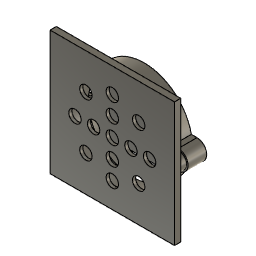
Speaker+Mount+Rev+1 (Autodesk Fusion 360 design; units mm, degrees)
Autodesk Fusion 360 part; units mm, degrees
sketch "Face" plane through (0, 0, 0) normal (0, 1, 0) x (1, 0, 0)
  line L0 (0, 0) -> (40, 0)
  line L1 (40, 0) -> (40, -40)
  line L2 (40, -40) -> (0, -40)
  line L3 (0, -40) -> (0, 0)
  circle A0 centre (20, -20) radius 14
  circle A1 centre (20, -20) radius 14.2
  circle A2 centre (20, -20) radius 14.7
  line L4 (0, -20) -> (40, -20)
  line L5 (5.5141, -22.5) -> (0.5141, -22.5)
  line L6 (0.5141, -22.5) -> (0.5141, -17.5)
  line L7 (0.5141, -17.5) -> (5.5141, -17.5)
  line L8 (5.5141, -17.5) -> (5.5141, -22.5)
  circle A3 centre (3.0141, -20) radius 2.5
  circle A4 centre (3.0141, -20) radius 1.5
  line L9 (34.4859, -22.5) -> (39.4859, -22.5)
  line L10 (39.4859, -22.5) -> (39.4859, -17.5)
  line L11 (39.4859, -17.5) -> (34.4859, -17.5)
  line L12 (34.4859, -17.5) -> (34.4859, -22.5)
  circle A5 centre (36.9859, -20) radius 2.5
  circle A6 centre (36.9859, -20) radius 1.5
  circle A7 centre (20, -32) radius 2
  circle A8 centre (28.4853, -28.4853) radius 2
  circle A9 centre (32, -20) radius 2
  circle A10 centre (28.4853, -11.5147) radius 2
  circle A11 centre (20, -8) radius 2
  circle A12 centre (11.5147, -11.5147) radius 2
  circle A13 centre (8, -20) radius 2
  circle A14 centre (11.5147, -28.4853) radius 2
  circle A15 centre (20, -26) radius 2
  circle A16 centre (26, -20) radius 2
  circle A17 centre (20, -14) radius 2
  circle A18 centre (14, -20) radius 2
  circle A19 centre (20, -20) radius 2
  dimension "d1" = 40
  dimension "d2" = 40
  dimension "d3" = 28
  dimension "d21" = 28.4
  dimension "d22" = 29.4
  dimension "d31" = 20
  dimension "d32" = 20
  dimension "d33" = 5
  dimension "d34" = 5
  dimension "d35" = 2.5
  dimension "d36" = 5
  dimension "d37" = 2.5
  dimension "d38" = 3
  dimension "d39" = 5
  dimension "d41" = 2.5
  dimension "d42" = 5
  dimension "d43" = 2.5
  dimension "d44" = 3
  dimension "d62" = 4
  dimension "d63" = 12
  dimension "d65" = 360
  dimension "d66" = 4
  dimension "d67" = 6
  dimension "d69" = 360
  dimension "d70" = 4
  constraint horizontal L0
  constraint vertical L1
  constraint horizontal L2
  constraint vertical L3
  constraint coincident L0.start L3.end
  constraint midpoint L3 L4.start
  constraint midpoint L1 L4.end
  constraint horizontal L5
  constraint vertical L6
  constraint horizontal L7
  constraint vertical L8
  constraint coincident A2 L5.start
  constraint coincident L4 A3.centre
  constraint concentric A3 A4
  constraint horizontal L9
  constraint vertical L10
  constraint horizontal L11
  constraint vertical L12
  constraint coincident A2 L9.start
  constraint coincident L4 A5.centre
  constraint concentric A5 A6
  constraint concentric A0 A19
  measures "d1" distance of L0.start L0.end
  measures "d2" distance of L0.start L2.end
  measures "d3" diameter of A0
  measures "d21" diameter of A1
  measures "d22" diameter of A2
  measures "d31" distance of L3 A0.centre
  measures "d32" distance of L0 A0.centre
  measures "d33" distance of L5.start L5.end
  measures "d34" distance of L5.start L7.end
  measures "d35" distance of L4 L7
  measures "d36" diameter of A3
  measures "d37" distance of L6 A3.centre
  measures "d38" diameter of A4
  measures "d39" distance of L9.start L9.end
  measures "d41" distance of L4 L9
  measures "d42" diameter of A5
  measures "d43" distance of L10 A5.centre
  measures "d44" diameter of A6
  measures "d62" diameter of A7
  measures "d63" distance of A0.centre A7.centre
  measures "d66" diameter of A15
  measures "d67" distance of A0.centre A15.centre
  measures "d70" diameter of A19
extrude "Extrude1" add sketch "Face" along normal blind 2 contours L0 L1 L3 A2 L4 L6 L7 L10 L11 | L1 L2 L3 A2 L4 L5 L6 L9 L10 | A2 L4 A3 A4 | L5 L6 A3 | L6 L7 A3 | A2 L4 A3 A4 | A2 L4 A5 A6 | L10 L11 A5 | A2 L4 A5 A6 | L9 L10 A5 | L4 A4 | L4 A4 | A2 L7 A3 | A2 L5 A3 | L4 A6 | L4 A6 | A2 L11 A5 | A2 L9 A5 makes body 1
extrude "Extrude2" add sketch "Face" along normal blind 6 contours A2 L8 A3 | A1 A2 L4 L8 L12 | A2 L4 A3 | A1 A2 L4 L8 L12 | A2 L8 A3 | A2 L4 A3 | A2 L12 A5 | A2 L4 A5 | A2 L12 A5 | A2 L4 A5 bodies 1
extrude "Extrude3" add sketch "Face" along normal blind 1 contours A0 A1 L4 | A0 A1 L4 | A14 | A7 | A8 | A0 L4 A9 A13 A16 A18 A19 | L4 A13 | A10 | A11 | A12 | A0 L4 A9 A13 A16 A18 A19 | L4 A13 | L4 A9 | L4 A9 | L4 A18 | L4 A18 | L4 A16 | L4 A16 | L4 A19 | L4 A19 | A15 | A17 bodies 1
extrude "Extrude4" add 1 faces at (5.5214, 6, 20.7303) along direction (0, 1, 0) blind 0.5 on bodies 1 bodies 1
extrude "Extrude5" add sketch "Face" along normal blind 6.5 contours A2 L4 A3 A4 | A2 L4 A3 A4 | A2 L4 A5 A6 | A2 L4 A5 A6 | A2 L7 A3 | A2 L5 A3 | A2 L11 A5 | A2 L9 A5 bodies 1
sketch "Back" plane through (0, 6.5, 0) normal (0, 1, 0) x (-1, 0, 0)
  circle A0 centre (-36.9859, 20) radius 1.5
  circle A1 centre (-3.0141, 20) radius 1.5
  circle A2 centre (-20, 20) radius 14.2
  arc A3 (-5.5141, 22.5) -> (-34.4859, 22.5) centre (-20, 20) ccw
  line L0 (-34.4859, 22.5) -> (-36.9859, 22.5)
  arc A4 (-36.9859, 22.5) -> (-36.9859, 17.5) centre (-36.9859, 20) ccw
  line L1 (-36.9859, 17.5) -> (-34.4859, 17.5)
  arc A5 (-34.4859, 17.5) -> (-5.5141, 17.5) centre (-20, 20) ccw
  line L2 (-5.5141, 17.5) -> (-3.0141, 17.5)
  arc A6 (-3.0141, 17.5) -> (-3.0141, 22.5) centre (-3.0141, 20) ccw
  line L3 (-3.0141, 22.5) -> (-5.5141, 22.5)
  circle A7 centre (-20, 20) radius 15
  circle A8 centre (-20, 20) radius 15.5
  circle A9 centre (-3.0141, 20) radius 2.65
  circle A10 centre (-36.9859, 20) radius 2.65
  circle A11 centre (-36.9859, 20) radius 3.15
  circle A12 centre (-3.0141, 20) radius 3.15
  line L4 (-36.9859, 20) -> (-35.1765, 20)
  line L5 (-35.1765, 20) -> (-35.1765, 23.15)
  line L6 (-35.1765, 23.15) -> (-36.9859, 23.15)
  line L7 (-36.9859, 23.15) -> (-36.9859, 20)
  line L8 (-36.9859, 20) -> (-35.1765, 20)
  line L9 (-35.1765, 20) -> (-35.1765, 16.85)
  line L10 (-35.1765, 16.85) -> (-36.9859, 16.85)
  line L11 (-36.9859, 16.85) -> (-36.9859, 20)
  line L12 (-36.9859, 20) -> (-35.0233, 20)
  line L13 (-35.0233, 20) -> (-35.0233, 22.65)
  line L14 (-35.0233, 22.65) -> (-36.9859, 22.65)
  line L15 (-36.9859, 22.65) -> (-36.9859, 20)
  line L16 (-36.9859, 17.35) -> (-35.1765, 17.35)
  line L17 (-35.1765, 17.35) -> (-35.1765, 20)
  line L18 (-35.1765, 20) -> (-36.9859, 20)
  line L19 (-36.9859, 20) -> (-36.9859, 17.35)
  line L20 (-3.0141, 23.15) -> (-5, 23.15)
  line L21 (-5, 23.15) -> (-5, 20)
  line L22 (-5, 20) -> (-3.0141, 20)
  line L23 (-3.0141, 20) -> (-3.0141, 23.15)
  line L24 (-3.0141, 22.65) -> (-5, 22.65)
  line L25 (-5, 22.65) -> (-5, 20)
  line L26 (-5, 20) -> (-3.0141, 20)
  line L27 (-3.0141, 20) -> (-3.0141, 22.65)
  line L28 (-3.0141, 16.85) -> (-5, 16.85)
  line L29 (-5, 16.85) -> (-5, 20)
  line L30 (-5, 20) -> (-3.0141, 20)
  line L31 (-3.0141, 20) -> (-3.0141, 16.85)
  line L32 (-5, 20) -> (-3.0141, 20)
  line L33 (-3.0141, 20) -> (-3.0141, 17.35)
  line L34 (-3.0141, 17.35) -> (-5, 17.35)
  line L35 (-5, 17.35) -> (-5, 20)
  line L36 (-35.1765, 17.35) -> (-34.6587, 17.35)
  line L37 (-34.6587, 17.35) -> (-34.6587, 16.8182)
  line L38 (-34.6587, 16.8182) -> (-35.1765, 16.8182)
  line L39 (-35.1765, 16.8182) -> (-35.1765, 17.35)
  line L40 (-35.0233, 22.65) -> (-34.6587, 22.65)
  line L41 (-34.6587, 22.65) -> (-34.6587, 23.1818)
  line L42 (-34.6587, 23.1818) -> (-35.0233, 23.1818)
  line L43 (-35.0233, 23.1818) -> (-35.0233, 22.65)
  line L44 (-5, 22.65) -> (-5.3413, 22.65)
  line L45 (-5.3413, 22.65) -> (-5.3413, 23.1818)
  line L46 (-5.3413, 23.1818) -> (-5, 23.1818)
  line L47 (-5, 23.1818) -> (-5, 22.65)
  line L48 (-5, 17.35) -> (-5.3413, 17.35)
  line L49 (-5.3413, 17.35) -> (-5.3413, 16.8182)
  line L50 (-5.3413, 16.8182) -> (-5, 16.8182)
  line L51 (-5, 16.8182) -> (-5, 17.35)
  dimension "d47" = 30
  dimension "d48" = 31
  dimension "d49" = 5.3
  dimension "d50" = 5.3
  dimension "d51" = 6.3
  dimension "d52" = 6.3
  dimension "d53" = 3.15
  dimension "d54" = 3.15
  dimension "d55" = 2.65
  constraint concentric A2 A7
  constraint concentric A7 A8
  constraint concentric A1 A9
  constraint concentric A0 A10
  constraint concentric A10 A11
  constraint concentric A9 A12
  constraint horizontal L4
  constraint vertical L5
  constraint horizontal L6
  constraint vertical L7
  constraint coincident A8 L5.end
  constraint coincident A0.centre A4.centre
  constraint horizontal L8
  constraint vertical L9
  constraint horizontal L10
  constraint vertical L11
  constraint coincident A8 L9.end
  constraint horizontal L12
  constraint vertical L13
  constraint horizontal L14
  constraint vertical L15
  constraint horizontal L16
  constraint vertical L17
  constraint horizontal L18
  constraint vertical L19
  constraint coincident L11 L16.start
  constraint coincident A10 L16.start
  constraint horizontal L20
  constraint vertical L21
  constraint horizontal L22
  constraint vertical L23
  constraint coincident A7 L21.end
  constraint coincident A12 L20.start
  constraint horizontal L24
  constraint vertical L25
  constraint horizontal L26
  constraint vertical L27
  constraint coincident A9 L24.start
  constraint coincident L23 L24.start
  constraint horizontal L28
  constraint vertical L29
  constraint horizontal L30
  constraint vertical L31
  constraint coincident A12 L28.start
  constraint horizontal L32
  constraint vertical L33
  constraint horizontal L34
  constraint vertical L35
  constraint coincident L31 L33.end
  constraint coincident A9 L33.end
  constraint horizontal L36
  constraint vertical L37
  constraint horizontal L38
  constraint vertical L39
  constraint coincident A7 L37.end
  constraint horizontal L40
  constraint vertical L41
  constraint horizontal L42
  constraint vertical L43
  constraint coincident A7 L41.end
  constraint horizontal L44
  constraint vertical L45
  constraint horizontal L46
  constraint vertical L47
  constraint coincident A7 L45.end
  constraint horizontal L48
  constraint vertical L49
  constraint horizontal L50
  constraint vertical L51
  constraint coincident A7 L49.end
  measures "d47" diameter of A7
  measures "d48" diameter of A8
  measures "d49" diameter of A9
  measures "d50" diameter of A10
  measures "d51" diameter of A11
  measures "d52" diameter of A12
  measures "d53" distance of A0.centre L6.end
  measures "d54" distance of A0.centre L10.end
  measures "d55" distance of A0.centre L14.end
extrude "Extrude6" add sketch "Back" against normal blind 1 separate body contours A0 A8 A10 L4 L8 L9 L12 L17 L18 | A0 A8 A10 L4 L5 L8 L12 L18 | A0 L0 A8 A10 L7 L15 | A0 L1 A8 A10 L11 L19 | A7 A10 L9 L12 L13 L17 | A10 L5 L12 L13 | A0 A4 L7 L11 L15 L19 | L0 A8 A10 | L0 A8 A10 L5 | L1 A8 A10 L9 L17 | L1 A8 A10 | L0 A10 A11 L5 L13 | L1 A7 A10 A11 L9 L17 | L0 A10 L7 L15 | A4 A10 L7 L11 L15 L19 | L0 A8 A11 L5 | L0 A8 A10 A11 L14 | L1 A10 L11 L19 | L1 A8 A10 A11 L16 | L1 A8 A11 L9 L17 | A7 A10 A11 L13 | L0 A11 L5 | A2 A7 A10 A11 | A7 A10 | L1 A11 L9 L17 | A10 A11 L7 L11 | A11 L7 L14 | A8 A11 L14 | A8 A11 L5 L14 | A11 L11 L16 | A8 A11 L9 L16 L17 | A8 A11 L16 | L0 A7 A11 L13 | L0 A11 L13 | L0 A11 L5 L13 L14 | A2 L1 A5 L2 A7 A11 A12 | L1 A7 A11 | L1 A7 A11 L9 L17 L36 | A8 A11 L6 L14 | A8 L5 L14 | A8 A11 L10 L16 | A8 L9 L16 L39 | A2 A3 L0 L3 A7 A11 A12 | L0 A7 L13 L40 | A7 A8 L5 L14 L20 L42 L43 L46 L47 | L1 A5 L2 A7 L36 L37 L48 L49 | A2 A11 A12 | A2 A11 | A7 A8 L9 L36 L38 L39 | A3 L0 L3 A7 L40 L41 L44 L45 | A7 L40 L42 L43 | A7 L36 L37 | A2 A12 | A2 A7 A9 A12 | A8 A12 L20 L24 | A8 L20 L21 L24 L47 | A7 A8 L28 L38 L50 L51 | A7 L40 L41 | L2 A7 A12 L29 L35 | A7 A9 A12 L29 L35 | A8 A12 L24 | L3 A8 A12 L21 L24 L25 | A12 L23 L24 | A9 A12 L23 L31 | A7 L21 L44 L46 L47 | A8 L28 L29 L34 L51 | A8 A12 L28 L34 | A7 A9 A12 L21 L25 | L3 A7 A12 L21 L25 | L2 A7 L29 L35 L48 | A7 L48 L49 | A7 L29 L48 L50 L51 | A7 A9 | A7 A9 L29 L35 | L2 A8 A9 A12 L29 L35 | L2 A12 L29 L35 | L3 A8 A9 A12 L24 | L3 A8 A12 | L3 A7 L21 L25 L44 | L3 A9 L23 L27 | A6 A9 L23 L27 L31 L33 | L2 A8 A12 L29 L34 L35 | A8 A12 L34 | A12 L31 L34 | A7 L44 L45 | A7 A9 L21 L25 | L3 A12 L21 L25 | L3 A8 A9 A12 L21 L25 | A1 A8 A9 L21 L22 L25 L26 L30 L32 | A1 A8 A9 L22 L26 L29 L30 L32 L35 | L2 A8 A12 | L3 A8 A9 | A1 L3 A8 A9 L23 L27 | A1 A6 L23 L27 L31 L33 | L2 A8 A9 A12 L34 | L2 A9 L31 L33 | L2 A8 A9 | A1 L2 A8 A9 L31 L33 makes body 2
extrude "Extrude7" add sketch "Back" along normal blind 5 contours A10 A11 L7 L11 | A11 L7 L14 | A11 L11 L16 | A8 A11 L6 L14 | A8 L5 L14 | A8 A11 L10 L16 | A8 L9 L16 L39 | A7 A8 L5 L14 L20 L42 L43 L46 L47 | A7 A8 L9 L36 L38 L39 | A7 L40 L42 L43 | A8 A12 L20 L24 | A8 L20 L21 L24 L47 | A7 A8 L28 L38 L50 L51 | A12 L23 L24 | A9 A12 L23 L31 | A7 L21 L44 L46 L47 | A8 L28 L29 L34 L51 | A8 A12 L28 L34 | A7 L29 L48 L50 L51 | A12 L31 L34 bodies 2
extrude "Extrude8" cut 2 faces at (36.6193, 2, 20.3401) (2.6277, 2, 20.3909) along direction (0, -1, 0) blind 1 on bodies 1 bodies 1
extrude "Extrude9" cut sketch "Face" along normal blind 1 contours A14 | A7 | A8 | L4 A13 | A10 | A11 | A12 | L4 A13 | L4 A9 | L4 A9 | L4 A18 | L4 A18 | L4 A16 | L4 A16 | L4 A19 | L4 A19 | A15 | A17 bodies 1
sketch "Wire Hole" plane through (0, 5.5, 0) normal (0, -1, 0) x (1, 0, 0)
  circle A0 centre (36.9859, 20) radius 1.5
  circle A1 centre (3.0141, 20) radius 1.5
  line L0 (4.8235, 23.15) -> (3.0141, 23.15)
  arc A2 (3.0141, 23.15) -> (3.0141, 16.85) centre (3.0141, 20) ccw
  line L1 (3.0141, 16.85) -> (4.8235, 16.85)
  arc A3 (4.8235, 16.85) -> (35.1765, 16.85) centre (20, 20) ccw
  line L2 (35.1765, 16.85) -> (36.9859, 16.85)
  arc A4 (36.9859, 16.85) -> (36.9859, 23.15) centre (36.9859, 20) ccw
  line L3 (36.9859, 23.15) -> (35.1765, 23.15)
  arc A5 (35.1765, 23.15) -> (4.8235, 23.15) centre (20, 20) ccw
  line L4 (15, 10) -> (25, 10)
  line L5 (25, 10) -> (25, 3)
  line L6 (25, 3) -> (15, 3)
  line L7 (15, 3) -> (15, 10)
  constraint horizontal L4
  constraint vertical L5
  constraint horizontal L6
  constraint vertical L7
extrude "Extrude11" cut sketch "Wire Hole" against normal blind 7 contours A3 L4 L5 L7 bodies 2
move_body "Move1" bodies 2 to x (-1, 0, 0) y (0, -1, 0) z (0, 0, 1) at (39.7283, 16, 0)
copy_body "Body->Comp1" bodies 1 removing the originals makes body 3 in component "Face"
copy_body "Body->Comp2" bodies 2 removing the originals makes body 4 in component "Back"
component "Face" placed x (1, 0, 0) y (0, 1, 0) z (0, 0, 1) at (0, 0, 0)
component "Back" placed x (1, 0, 0) y (0, 1, 0) z (0, 0, 1) at (0, 0, 0)
named bodies: "Face", "Back"
